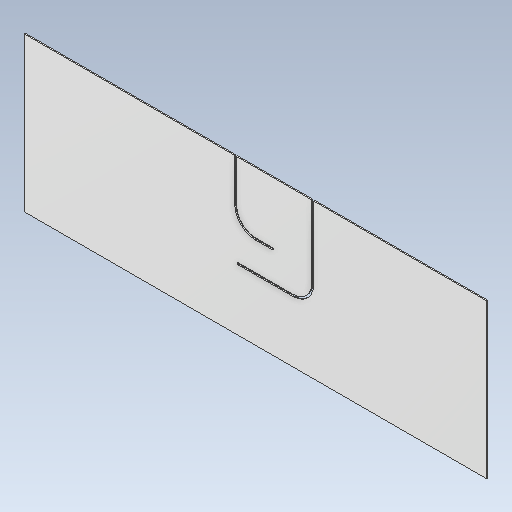
# Autodesk Inventor part: btwnFerriteAndCoil
Saved by Autodesk Inventor 2021 (Build 250183000, 183)
## iProperties
Created: 2022-01-22
Part Number: btwnFerriteAndCoil
Material: LCP Plastic
Document SubType Name: Modeling
Designer: avan411
Density: 1.626 g/cm^3
Appearance: Smooth - White
Author: avan411
Autodesk Inventor part; units mm, degrees
ref_plane "YZ Plane" through (0, 0, 0) normal (1, 0, 0) x (0, 1, 0)
ref_plane "XZ Plane" through (0, 0, 0) normal (0, 1, 0) x (-1, 0, 0)
ref_plane "XY Plane" through (0, 0, 0) normal (0, 0, 1) x (1, 0, 0)
sketch "Sketch1" plane through (0, 0, 0) normal (0, 0, 1) x (1, 0, 0)
  line L0 (-525, 175) -> (525, 175) projected
  line L1 (-525, -175) -> (-525, 175) projected
  line L2 (525, -175) -> (-525, -175) projected
  line L3 (525, 175) -> (525, -175) projected
  arc A0 (-434.5, -36.45) -> (-475.35, -77.3) centre (-434.5, -77.3) ccw projected
  line L4 (-475.35, -85.5) -> (-475.35, -77.3) projected
  arc A1 (-475.35, -85.5) -> (-434.5, -126.35) centre (-434.5, -85.5) ccw projected
  line L5 (434.5, -126.35) -> (-434.5, -126.35) projected
  arc A2 (434.5, -126.35) -> (475.35, -85.5) centre (434.5, -85.5) ccw projected
  line L6 (475.35, -65.8667) -> (475.35, -85.5) projected
  arc A3 (475.35, -65.8667) -> (434.5, -25.0167) centre (434.5, -65.8667) ccw projected
  line L7 (-445.75, -25.0167) -> (434.5, -25.0167) projected
  arc A4 (-445.75, -25.0167) -> (-486.6, -65.8667) centre (-445.75, -65.8667) ccw projected
  line L8 (-486.6, -96.25) -> (-486.6, -65.8667) projected
  arc A5 (-486.6, -96.25) -> (-445.75, -137.1) centre (-445.75, -96.25) ccw projected
  line L9 (445.75, -137.1) -> (-445.75, -137.1) projected
  arc A6 (445.75, -137.1) -> (486.6, -96.25) centre (445.75, -96.25) ccw projected
  line L10 (486.6, -54.4333) -> (486.6, -96.25) projected
  arc A7 (486.6, -54.4333) -> (445.75, -13.5833) centre (445.75, -54.4333) ccw projected
  line L11 (-457, -13.5833) -> (445.75, -13.5833) projected
  arc A8 (-457, -13.5833) -> (-497.85, -54.4333) centre (-457, -54.4333) ccw projected
  line L12 (-497.85, -107) -> (-497.85, -54.4333) projected
  arc A9 (-497.85, -107) -> (-457, -147.85) centre (-457, -107) ccw projected
  line L13 (457, -147.85) -> (-457, -147.85) projected
  arc A10 (457, -147.85) -> (497.85, -107) centre (457, -107) ccw projected
  line L14 (497.85, -43) -> (497.85, -107) projected
  arc A11 (497.85, -43) -> (457, -2.15) centre (457, -43) ccw projected
  line L15 (-457, -2.15) -> (457, -2.15) projected
  arc A12 (-502.15, 43) -> (-457, -2.15) centre (-457, 43) ccw projected
  line L16 (-502.15, 107) -> (-502.15, 43) projected
  arc A13 (-457, 152.15) -> (-502.15, 107) centre (-457, 107) ccw projected
  line L17 (457, 152.15) -> (-457, 152.15) projected
  arc A14 (502.15, 107) -> (457, 152.15) centre (457, 107) ccw projected
  line L18 (502.15, 54.4333) -> (502.15, 107) projected
  arc A15 (457, 9.2833) -> (502.15, 54.4333) centre (457, 54.4333) ccw projected
  line L19 (-445.75, 9.2833) -> (457, 9.2833) projected
  arc A16 (-490.9, 54.4333) -> (-445.75, 9.2833) centre (-445.75, 54.4333) ccw projected
  line L20 (-490.9, 96.25) -> (-490.9, 54.4333) projected
  arc A17 (-445.75, 141.4) -> (-490.9, 96.25) centre (-445.75, 96.25) ccw projected
  line L21 (445.75, 141.4) -> (-445.75, 141.4) projected
  arc A18 (490.9, 96.25) -> (445.75, 141.4) centre (445.75, 96.25) ccw projected
  line L22 (490.9, 65.8667) -> (490.9, 96.25) projected
  arc A19 (445.75, 20.7167) -> (490.9, 65.8667) centre (445.75, 65.8667) ccw projected
  line L23 (-434.5, 20.7167) -> (445.75, 20.7167) projected
  arc A20 (-479.65, 65.8667) -> (-434.5, 20.7167) centre (-434.5, 65.8667) ccw projected
  line L24 (-479.65, 85.5) -> (-479.65, 65.8667) projected
  arc A21 (-434.5, 130.65) -> (-479.65, 85.5) centre (-434.5, 85.5) ccw projected
  line L25 (434.5, 130.65) -> (-434.5, 130.65) projected
  arc A22 (479.65, 85.5) -> (434.5, 130.65) centre (434.5, 85.5) ccw projected
  line L26 (479.65, 77.3) -> (479.65, 85.5) projected
  arc A23 (434.5, 32.15) -> (479.65, 77.3) centre (434.5, 77.3) ccw projected
  line L27 (0, 32.15) -> (434.5, 32.15) projected
  line L28 (0, 36.45) -> (0, 32.15) projected
  line L29 (434.5, 36.45) -> (0, 36.45) projected
  arc A24 (434.5, 36.45) -> (475.35, 77.3) centre (434.5, 77.3) ccw projected
  line L30 (475.35, 85.5) -> (475.35, 77.3) projected
  arc A25 (475.35, 85.5) -> (434.5, 126.35) centre (434.5, 85.5) ccw projected
  line L31 (-434.5, 126.35) -> (434.5, 126.35) projected
  arc A26 (-434.5, 126.35) -> (-475.35, 85.5) centre (-434.5, 85.5) ccw projected
  line L32 (-475.35, 65.8667) -> (-475.35, 85.5) projected
  arc A27 (-475.35, 65.8667) -> (-434.5, 25.0167) centre (-434.5, 65.8667) ccw projected
  line L33 (445.75, 25.0167) -> (-434.5, 25.0167) projected
  arc A28 (445.75, 25.0167) -> (486.6, 65.8667) centre (445.75, 65.8667) ccw projected
  line L34 (486.6, 96.25) -> (486.6, 65.8667) projected
  arc A29 (486.6, 96.25) -> (445.75, 137.1) centre (445.75, 96.25) ccw projected
  line L35 (-445.75, 137.1) -> (445.75, 137.1) projected
  arc A30 (-445.75, 137.1) -> (-486.6, 96.25) centre (-445.75, 96.25) ccw projected
  line L36 (-486.6, 54.4333) -> (-486.6, 96.25) projected
  arc A31 (-486.6, 54.4333) -> (-445.75, 13.5833) centre (-445.75, 54.4333) ccw projected
  line L37 (457, 13.5833) -> (-445.75, 13.5833) projected
  arc A32 (457, 13.5833) -> (497.85, 54.4333) centre (457, 54.4333) ccw projected
  line L38 (497.85, 107) -> (497.85, 54.4333) projected
  arc A33 (497.85, 107) -> (457, 147.85) centre (457, 107) ccw projected
  line L39 (-457, 147.85) -> (457, 147.85) projected
  arc A34 (-457, 147.85) -> (-497.85, 107) centre (-457, 107) ccw projected
  line L40 (-497.85, 43) -> (-497.85, 107) projected
  arc A35 (-497.85, 43) -> (-457, 2.15) centre (-457, 43) ccw projected
  line L41 (457, 2.15) -> (-457, 2.15) projected
  arc A36 (502.15, -43) -> (457, 2.15) centre (457, -43) ccw projected
  line L42 (502.15, -107) -> (502.15, -43) projected
  arc A37 (457, -152.15) -> (502.15, -107) centre (457, -107) ccw projected
  line L43 (-457, -152.15) -> (457, -152.15) projected
  arc A38 (-502.15, -107) -> (-457, -152.15) centre (-457, -107) ccw projected
  line L44 (-502.15, -54.4333) -> (-502.15, -107) projected
  arc A39 (-457, -9.2833) -> (-502.15, -54.4333) centre (-457, -54.4333) ccw projected
  line L45 (445.75, -9.2833) -> (-457, -9.2833) projected
  arc A40 (490.9, -54.4333) -> (445.75, -9.2833) centre (445.75, -54.4333) ccw projected
  line L46 (490.9, -96.25) -> (490.9, -54.4333) projected
  arc A41 (445.75, -141.4) -> (490.9, -96.25) centre (445.75, -96.25) ccw projected
  line L47 (-445.75, -141.4) -> (445.75, -141.4) projected
  arc A42 (-490.9, -96.25) -> (-445.75, -141.4) centre (-445.75, -96.25) ccw projected
  line L48 (-490.9, -65.8667) -> (-490.9, -96.25) projected
  arc A43 (-445.75, -20.7167) -> (-490.9, -65.8667) centre (-445.75, -65.8667) ccw projected
  line L49 (434.5, -20.7167) -> (-445.75, -20.7167) projected
  arc A44 (479.65, -65.8667) -> (434.5, -20.7167) centre (434.5, -65.8667) ccw projected
  line L50 (479.65, -85.5) -> (479.65, -65.8667) projected
  arc A45 (434.5, -130.65) -> (479.65, -85.5) centre (434.5, -85.5) ccw projected
  line L51 (-434.5, -130.65) -> (434.5, -130.65) projected
  arc A46 (-479.65, -85.5) -> (-434.5, -130.65) centre (-434.5, -85.5) ccw projected
  line L52 (-479.65, -77.3) -> (-479.65, -85.5) projected
  arc A47 (-434.5, -32.15) -> (-479.65, -77.3) centre (-434.5, -77.3) ccw projected
  line L53 (0, -32.15) -> (-434.5, -32.15) projected
  line L54 (0, -36.45) -> (0, -32.15) projected
  line L55 (-434.5, -36.45) -> (0, -36.45) projected
  line L56 (-525, 175) -> (525, 175) projected
  line L57 (-525, -175) -> (-525, 175) projected
  line L58 (525, -175) -> (-525, -175) projected
  line L59 (525, 175) -> (525, -175) projected
  arc A48 (-434.5, -36.45) -> (-475.35, -77.3) centre (-434.5, -77.3) ccw projected
  line L60 (-475.35, -85.5) -> (-475.35, -77.3) projected
  arc A49 (-475.35, -85.5) -> (-434.5, -126.35) centre (-434.5, -85.5) ccw projected
  line L61 (434.5, -126.35) -> (-434.5, -126.35) projected
  arc A50 (434.5, -126.35) -> (475.35, -85.5) centre (434.5, -85.5) ccw projected
  line L62 (475.35, -65.8667) -> (475.35, -85.5) projected
  arc A51 (475.35, -65.8667) -> (434.5, -25.0167) centre (434.5, -65.8667) ccw projected
  line L63 (-445.75, -25.0167) -> (434.5, -25.0167) projected
  arc A52 (-445.75, -25.0167) -> (-486.6, -65.8667) centre (-445.75, -65.8667) ccw projected
  line L64 (-486.6, -96.25) -> (-486.6, -65.8667) projected
  arc A53 (-486.6, -96.25) -> (-445.75, -137.1) centre (-445.75, -96.25) ccw projected
  line L65 (445.75, -137.1) -> (-445.75, -137.1) projected
  arc A54 (445.75, -137.1) -> (486.6, -96.25) centre (445.75, -96.25) ccw projected
  line L66 (486.6, -54.4333) -> (486.6, -96.25) projected
  arc A55 (486.6, -54.4333) -> (445.75, -13.5833) centre (445.75, -54.4333) ccw projected
  line L67 (-457, -13.5833) -> (445.75, -13.5833) projected
  arc A56 (-457, -13.5833) -> (-497.85, -54.4333) centre (-457, -54.4333) ccw projected
  line L68 (-497.85, -107) -> (-497.85, -54.4333) projected
  arc A57 (-497.85, -107) -> (-457, -147.85) centre (-457, -107) ccw projected
  line L69 (457, -147.85) -> (-457, -147.85) projected
  arc A58 (457, -147.85) -> (497.85, -107) centre (457, -107) ccw projected
  line L70 (497.85, -43) -> (497.85, -107) projected
  arc A59 (497.85, -43) -> (457, -2.15) centre (457, -43) ccw projected
  line L71 (-457, -2.15) -> (457, -2.15) projected
  arc A60 (-502.15, 43) -> (-457, -2.15) centre (-457, 43) ccw projected
  line L72 (-502.15, 107) -> (-502.15, 43) projected
  arc A61 (-457, 152.15) -> (-502.15, 107) centre (-457, 107) ccw projected
  line L73 (457, 152.15) -> (-457, 152.15) projected
  arc A62 (502.15, 107) -> (457, 152.15) centre (457, 107) ccw projected
  line L74 (502.15, 54.4333) -> (502.15, 107) projected
  arc A63 (457, 9.2833) -> (502.15, 54.4333) centre (457, 54.4333) ccw projected
  line L75 (-445.75, 9.2833) -> (457, 9.2833) projected
  arc A64 (-490.9, 54.4333) -> (-445.75, 9.2833) centre (-445.75, 54.4333) ccw projected
  line L76 (-490.9, 96.25) -> (-490.9, 54.4333) projected
  arc A65 (-445.75, 141.4) -> (-490.9, 96.25) centre (-445.75, 96.25) ccw projected
  line L77 (445.75, 141.4) -> (-445.75, 141.4) projected
  arc A66 (490.9, 96.25) -> (445.75, 141.4) centre (445.75, 96.25) ccw projected
  line L78 (490.9, 65.8667) -> (490.9, 96.25) projected
  arc A67 (445.75, 20.7167) -> (490.9, 65.8667) centre (445.75, 65.8667) ccw projected
  line L79 (-434.5, 20.7167) -> (445.75, 20.7167) projected
  arc A68 (-479.65, 65.8667) -> (-434.5, 20.7167) centre (-434.5, 65.8667) ccw projected
  line L80 (-479.65, 85.5) -> (-479.65, 65.8667) projected
  arc A69 (-434.5, 130.65) -> (-479.65, 85.5) centre (-434.5, 85.5) ccw projected
  line L81 (434.5, 130.65) -> (-434.5, 130.65) projected
  arc A70 (479.65, 85.5) -> (434.5, 130.65) centre (434.5, 85.5) ccw projected
  line L82 (479.65, 77.3) -> (479.65, 85.5) projected
  arc A71 (434.5, 32.15) -> (479.65, 77.3) centre (434.5, 77.3) ccw projected
  line L83 (0, 32.15) -> (434.5, 32.15) projected
  line L84 (0, 36.45) -> (0, 32.15) projected
  line L85 (434.5, 36.45) -> (0, 36.45) projected
  arc A72 (434.5, 36.45) -> (475.35, 77.3) centre (434.5, 77.3) ccw projected
  line L86 (475.35, 85.5) -> (475.35, 77.3) projected
  arc A73 (475.35, 85.5) -> (434.5, 126.35) centre (434.5, 85.5) ccw projected
  line L87 (-434.5, 126.35) -> (434.5, 126.35) projected
  arc A74 (-434.5, 126.35) -> (-475.35, 85.5) centre (-434.5, 85.5) ccw projected
  line L88 (-475.35, 65.8667) -> (-475.35, 85.5) projected
  arc A75 (-475.35, 65.8667) -> (-434.5, 25.0167) centre (-434.5, 65.8667) ccw projected
  line L89 (445.75, 25.0167) -> (-434.5, 25.0167) projected
  arc A76 (445.75, 25.0167) -> (486.6, 65.8667) centre (445.75, 65.8667) ccw projected
  line L90 (486.6, 96.25) -> (486.6, 65.8667) projected
  arc A77 (486.6, 96.25) -> (445.75, 137.1) centre (445.75, 96.25) ccw projected
  line L91 (-445.75, 137.1) -> (445.75, 137.1) projected
  arc A78 (-445.75, 137.1) -> (-486.6, 96.25) centre (-445.75, 96.25) ccw projected
  line L92 (-486.6, 54.4333) -> (-486.6, 96.25) projected
  arc A79 (-486.6, 54.4333) -> (-445.75, 13.5833) centre (-445.75, 54.4333) ccw projected
  line L93 (457, 13.5833) -> (-445.75, 13.5833) projected
  arc A80 (457, 13.5833) -> (497.85, 54.4333) centre (457, 54.4333) ccw projected
  line L94 (497.85, 107) -> (497.85, 54.4333) projected
  arc A81 (497.85, 107) -> (457, 147.85) centre (457, 107) ccw projected
  line L95 (-457, 147.85) -> (457, 147.85) projected
  arc A82 (-457, 147.85) -> (-497.85, 107) centre (-457, 107) ccw projected
  line L96 (-497.85, 43) -> (-497.85, 107) projected
  arc A83 (-497.85, 43) -> (-457, 2.15) centre (-457, 43) ccw projected
  line L97 (457, 2.15) -> (-457, 2.15) projected
  arc A84 (502.15, -43) -> (457, 2.15) centre (457, -43) ccw projected
  line L98 (502.15, -107) -> (502.15, -43) projected
  arc A85 (457, -152.15) -> (502.15, -107) centre (457, -107) ccw projected
  line L99 (-457, -152.15) -> (457, -152.15) projected
  arc A86 (-502.15, -107) -> (-457, -152.15) centre (-457, -107) ccw projected
  line L100 (-502.15, -54.4333) -> (-502.15, -107) projected
  arc A87 (-457, -9.2833) -> (-502.15, -54.4333) centre (-457, -54.4333) ccw projected
  line L101 (445.75, -9.2833) -> (-457, -9.2833) projected
  arc A88 (490.9, -54.4333) -> (445.75, -9.2833) centre (445.75, -54.4333) ccw projected
  line L102 (490.9, -96.25) -> (490.9, -54.4333) projected
  arc A89 (445.75, -141.4) -> (490.9, -96.25) centre (445.75, -96.25) ccw projected
  line L103 (-445.75, -141.4) -> (445.75, -141.4) projected
  arc A90 (-490.9, -96.25) -> (-445.75, -141.4) centre (-445.75, -96.25) ccw projected
  line L104 (-490.9, -65.8667) -> (-490.9, -96.25) projected
  arc A91 (-445.75, -20.7167) -> (-490.9, -65.8667) centre (-445.75, -65.8667) ccw projected
  line L105 (434.5, -20.7167) -> (-445.75, -20.7167) projected
  arc A92 (479.65, -65.8667) -> (434.5, -20.7167) centre (434.5, -65.8667) ccw projected
  line L106 (479.65, -85.5) -> (479.65, -65.8667) projected
  arc A93 (434.5, -130.65) -> (479.65, -85.5) centre (434.5, -85.5) ccw projected
  line L107 (-434.5, -130.65) -> (434.5, -130.65) projected
  arc A94 (-479.65, -85.5) -> (-434.5, -130.65) centre (-434.5, -85.5) ccw projected
  line L108 (-479.65, -77.3) -> (-479.65, -85.5) projected
  arc A95 (-434.5, -32.15) -> (-479.65, -77.3) centre (-434.5, -77.3) ccw projected
  line L109 (0, -32.15) -> (-434.5, -32.15) projected
  line L110 (0, -36.45) -> (0, -32.15) projected
  line L111 (-434.5, -36.45) -> (0, -36.45) projected
  line L112 (0, -32.15) -> (0, 10.85) construction
  line L113 (18.1865, 10.85) -> (0, 10.85) construction
  line L114 (0, -36.45) -> (0, 10.85) construction
  line L115 (25.3634, 10.85) -> (0, 10.85) construction
  arc A96 (-43, 79.45) -> (0, 36.45) centre (0, 79.45) ccw
  line L116 (0, 36.45) -> (0, 79.45) construction
  line L117 (-43, 79.45) -> (0, 79.45) construction
  arc A97 (-47.3, 79.45) -> (0, 32.15) centre (0, 79.45) ccw
  line L118 (0, 32.15) -> (0, 79.45) construction
  line L119 (-47.3, 79.45) -> (0, 79.45) construction
  line L120 (-43, 79.45) -> (-43, 175)
  line L121 (-47.3, 79.45) -> (-47.3, 175)
  line L122 (85.0479, 2.11) -> (85.0479, -106.33) projected
  line L123 (0, -36.45) -> (85.0479, -36.45)
  line L124 (0, -32.15) -> (85.0479, -32.15)
  arc A98 (85.0479, -32.15) -> (128.0479, 10.85) centre (85.0479, 10.85) ccw
  line L125 (85.0479, -32.15) -> (85.0479, 10.85) construction
  line L126 (128.0479, 10.85) -> (85.0479, 10.85) construction
  arc A99 (85.0479, -36.45) -> (132.3479, 10.85) centre (85.0479, 10.85) ccw
  line L127 (85.0479, -36.45) -> (85.0479, 10.85) construction
  line L128 (132.3479, 10.85) -> (85.0479, 10.85) construction
  line L129 (128.0479, 10.85) -> (128.0479, 175)
  line L130 (132.3479, 10.85) -> (132.3479, 175)
  line L131 (0, 36.45) -> (0, 32.15)
  line L132 (0, -36.45) -> (0, -32.15)
  line L133 (-40, -32.15) -> (-40, -36.45)
  line L134 (40, 36.45) -> (40, 32.15)
  point P0 (0, 0)
  point P1 (128.0479, 175)
  point P2 (132.3479, 175)
  dimension "d4" = 90
  dimension "d6" = 90
  dimension "d7" = 43
  dimension "d8" = 90
  dimension "d9" = 47.3
  dimension "d10" = 90
  dimension "d11" = 43
  dimension "d12" = 90
  dimension "d13" = 47.3
  dimension "d14" = 90
  dimension "d17" = 40
  dimension "d18" = 40
  constraints: 44 end point, 10 point on line, 8 point on circle, 7 perpendicular, 4 centre point, 4 tangent, 3 equal length
  measures "d4" angle of L112 L113
  measures "d6" angle of L114 L115
  measures "d7" radius of A96
  measures "d8" angle of L117 L116
  measures "d9" radius of A97
  measures "d10" angle of L119 L118
  measures "d11" radius of A98
  measures "d12" angle of L125 L126
  measures "d13" radius of A99
  measures "d14" angle of L127 L128
  measures "d17" distance between parallel lines of L133 L110
  measures "d18" distance between parallel lines of L118 L134
extrude "Extrusion1" add sketch "Sketch1" along normal blind 2.5 contours L0 L121 L17 A13 L16 A12 L15 L122 L45 A39 L44 A38 L43 A37 L42 A36 L41 A99 L19 A15 L18 A14 L130 L3 L2 L1 | L0 L129 L17 L120 | L121 L39 A34 L40 A35 L41 A98 L15 A12 L16 A13 L17 | L17 L129 L39 L120 | L121 L21 A17 L20 A16 L19 A98 L41 A35 L40 A34 L39 | L39 L129 L21 L120 | L121 L35 A30 L36 A31 L37 L129 A98 L19 A16 L20 A17 L21 | L17 A14 L18 A15 L19 A99 L130 L37 A32 L38 A33 L39 | L21 L129 L35 L120 | L121 L25 A21 L24 A20 L23 L129 L37 A31 L36 A30 L35 | L39 A33 L38 A32 L37 L130 L23 A19 L22 A18 L21 | L35 L129 L25 L120 | L121 L31 A26 L32 A27 L33 L129 L23 A20 L24 A21 L25 | L21 A18 L22 A19 L23 L130 L33 A28 L34 A29 L35 | L25 L129 L31 L120 | L15 A98 L45 L122 | L121 A97 L27 L129 L33 A27 L32 A26 L31 | L35 A29 L34 A28 L33 L130 L27 A23 L26 A22 L25 | L31 L129 L29 A96 L120 | L122 L11 A8 L12 A9 L13 A10 L14 A11 L15 A99 L41 A36 L42 A37 L43 A38 L44 A39 L45 | L45 A98 L11 L122 | L25 A22 L26 A23 L27 L130 L29 A24 L30 A25 L31 | L15 A11 L14 A10 L13 A9 L12 A8 L11 L122 L49 A43 L48 A42 L47 A41 L46 A40 L45 A99 | L11 A98 L49 L122 | L31 A25 L30 A24 L29 L130 | L129 L27 L134 L29 | L45 A40 L46 A41 L47 A42 L48 A43 L49 L122 L7 A4 L8 A5 L9 A6 L10 A7 L11 A99 | L49 A98 L7 L122 | L11 A7 L10 A6 L9 A5 L8 A4 L7 L122 L124 L53 A47 L52 A46 L51 A45 L50 A44 L49 A99 | L7 A98 L122 | L49 A44 L50 A45 L51 A46 L52 A47 L53 L133 L55 A0 L4 A1 L5 A2 L6 A3 L7 A99 | L7 A3 L6 A2 L5 A1 L4 A0 L55 L123 A99
body "Solid1"
